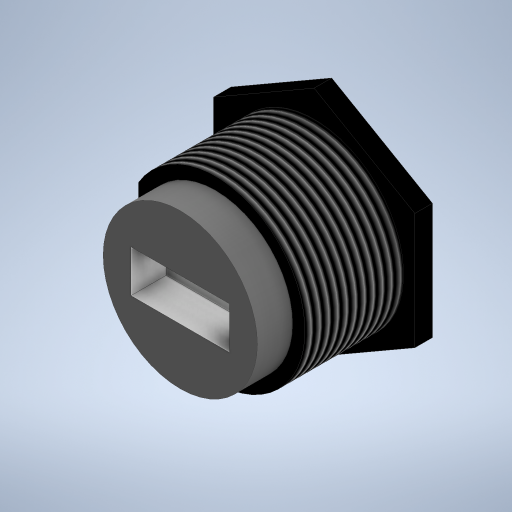
# Autodesk Inventor part: RS PRO USB 2.0 Cable, Female USB A to Male USB A USB Extension Cable, 200mm
Saved by Autodesk Inventor 2023 (Build 270158000, 158)
## iProperties
Created: 2023-04-24
Part Number: RS PRO USB 2.0 Cable, Female USB A to Male USB A USB Extension Cable, 200mm
Material: Generic
Document SubType Name: Modeling
Designer: Louis
Density: 1 g/cm^3
Appearance: Default
Author: Louis
Autodesk Inventor part; units mm, degrees
ref_plane "YZ Plane" through (0, 0, 0) normal (1, 0, 0) x (0, 1, 0)
ref_plane "XZ Plane" through (0, 0, 0) normal (0, 1, 0) x (-1, 0, 0)
ref_plane "XY Plane" through (0, 0, 0) normal (0, 0, 1) x (1, 0, 0)
sketch "Sketch1" plane through (0, 0, 0) normal (0, 0, 1) x (1, 0, 0)
  circle A0 centre (0, 0) radius 12.7
  line L0 (-10.95, 6.4333) -> (-10.95, -6.4333)
  dimension "d0" = 25.4
  dimension "d1" = 23.65
  constraints: 2 end point, 2 point on circle, 1 centre point, 1 coincident, 1 vertical
  measures "d0" diameter of A0
extrude "Extrusion1" add sketch "Sketch1" along normal blind 19 contours A0 L0 picked at (-3.0667, 0)
sketch "Sketch2" plane through (0, 0, 0) normal (0, 0, -1) x (-1, 0, 0)
  line L0 (0, 16.5122) -> (14.3, 8.2561)
  line L1 (14.3, 8.2561) -> (14.3, -8.2561)
  line L2 (14.3, -8.2561) -> (0, -16.5122)
  line L3 (0, -16.5122) -> (-14.3, -8.2561)
  line L4 (-14.3, -8.2561) -> (-14.3, 8.2561)
  line L5 (-14.3, 8.2561) -> (0, 16.5122)
  point P0 (0, 0)
  point P1 (0, 0)
  dimension "d5" = 28.6
  constraints: 12 end point, 1 coincident, 13 other
  measures "d5" distance between parallel lines of L1 L4
extrude "Extrusion2" add sketch "Sketch2" along normal blind 2.5
sketch "Sketch3" plane through (0, 0, 19) normal (0, 0, 1) x (1, 0, 0)
  circle A0 centre (0, 0) radius 10.95
  arc A1 (-10.95, -6.4333) -> (-10.95, 6.4333) centre (0, 0) ccw projected
  line L0 (-10.95, 6.4333) -> (-10.95, -6.4333) projected
  point P0 (-10.95, 0)
  constraints: 1 centre point, 1 coincident
extrude "Extrusion3" cut sketch "Sketch3" against normal blind 5
sketch "Sketch4" plane through (0, 0, 19) normal (0, 0, 1) x (1, 0, 0)
  line L0 (-7, 3) -> (7, 3)
  line L1 (7, 3) -> (7, -3)
  line L2 (7, -3) -> (-7, -3)
  line L3 (-7, -3) -> (-7, 3)
  point P0 (0, 0)
  point P1 (7, 0)
  point P2 (0, 3)
  dimension "d10" = 14
  dimension "d11" = 6
  constraints: 8 end point, 2 midpoint, 2 parallel, 1 horizontal, 1 horizontal alignment, 1 perpendicular, 1 vertical alignment
  measures "d10" distance of L0.start L0.end
  measures "d11" distance of L0.end L1.end
extrude "Extrusion4" cut sketch "Sketch4" against normal blind 5
thread "Thread1" size "1-20 UNEF" class "2A" standard "ANSI Unified Screw Threads" full length
body "Solid1"
